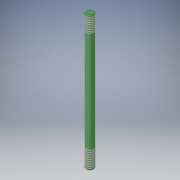
# Autodesk Inventor part: studs
Saved by Autodesk Inventor 2017 (Build 210142000, 142)
## iProperties
Created: 2019-11-21
Part Number: studs
Material: Silver
Document SubType Name: Modeling
Designer: 722650
Density: 10.49 g/cm^3
Appearance: Smooth - Dark Forest Green
Author: 722650
Autodesk Inventor part; units mm, degrees
ref_plane "YZ Plane" through (0, 0, 0) normal (1, 0, 0) x (0, 1, 0)
ref_plane "XZ Plane" through (0, 0, 0) normal (0, 1, 0) x (-1, 0, 0)
ref_plane "XY Plane" through (0, 0, 0) normal (0, 0, 1) x (1, 0, 0)
sketch "Sketch1" plane through (0, 0, 0) normal (0, 1, 0) x (-1, 0, 0)
  circle A0 centre (0, 0) radius 1.0922
  dimension "d0" = 2.1844
  constraints: 1 centre point, 1 coincident
  measures "d0" diameter of A0
extrude "Extrusion1" add sketch "Sketch1" along normal blind 39.6875
thread "Thread1" size "2-56 UNC" class "2A" standard "ANSI Unified Screw Threads" length 4.7625
thread "Thread2" size "2-56 UNC" class "2A" standard "ANSI Unified Screw Threads" length 5.5563
fillet "Fillet1" radius 0.3175 2 edges at (1.0922, 39.6875, 0) (1.0922, 0, 0)
body "Solid1"
